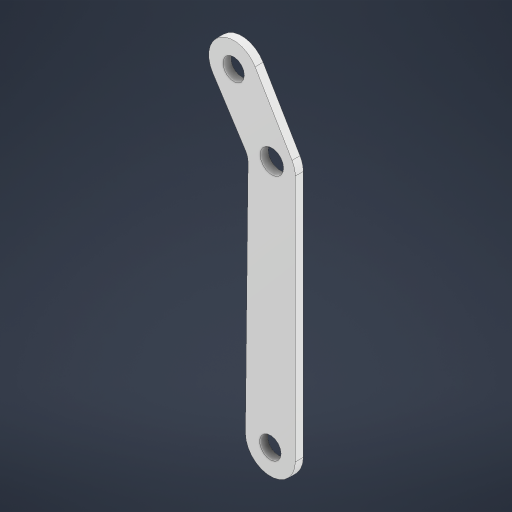
# Autodesk Inventor part: pneumaticwingplexi
Saved by Autodesk Inventor 2023 (Build 270158000, 158)
## iProperties
Created: 2023-08-07
Part Number: pneumaticwingplexi
Material: Generic
Document SubType Name: Modeling
Designer: srbel
Density: 1 g/cm^3
Appearance: Smooth - White
Mass: 1.20002 g
Surface Area: 18.206 cm^2
Volume: 1.20002 cm^3
Author: srbel
Autodesk Inventor part; units mm, degrees
ref_plane "YZ Plane" through (0, 0, 0) normal (1, 0, 0) x (0, 1, 0)
ref_plane "XZ Plane" through (0, 0, 0) normal (0, 1, 0) x (-1, 0, 0)
ref_plane "XY Plane" through (0, 0, 0) normal (0, 0, 1) x (1, 0, 0)
sketch "Sketch2" plane through (0, 0, 0) normal (0, 0, 1) x (1, 0, 0)
  circle A0 centre (-4.7681, 50.6628) radius 2.39
  circle A1 centre (-4.7681, 50.6628) radius 2.39
  circle A2 centre (-5.08, 0) radius 2.1844
  circle A3 centre (-12.5662, 63.0568) radius 2.1844
  arc A4 (-10.1597, 0.0569) -> (0, 0) centre (-5.08, 0) ccw
  arc A5 (-8.1919, 65.6399) -> (-16.8387, 60.3087) centre (-12.5662, 63.0568) ccw
  line L0 (-16.8387, 60.3087) -> (-10.1261, 49.8724)
  line L1 (-0.6665, 52.8961) -> (-8.1919, 65.6399)
  line L2 (0, 0) -> (0, 50.4566)
  arc A6 (0, 50.4566) -> (-0.6665, 52.8961) centre (-4.7976, 50.4566) ccw
  line L3 (-9.6216, 48.1193) -> (-10.1597, 0.0569)
  arc A7 (-9.6216, 48.1193) -> (-10.1261, 49.8724) centre (-12.7964, 48.1549) ccw
  circle A8 centre (-12.5662, 63.0568) radius 2.1844
  circle A9 centre (-5.08, 0) radius 2.1844
  arc A10 (-10.1597, 0.0569) -> (0, 0) centre (-5.08, 0) ccw
  line L4 (-10.1597, 0.0569) -> (-9.6216, 48.1193)
  line L5 (-10.1261, 49.8724) -> (-16.8387, 60.3087)
  arc A11 (-9.6216, 48.1193) -> (-10.1261, 49.8724) centre (-12.7964, 48.1549) ccw
  arc A12 (-8.1919, 65.6399) -> (-16.8387, 60.3087) centre (-12.5662, 63.0568) ccw
  line L6 (-8.1919, 65.6399) -> (-0.6665, 52.8961)
  constraints: 14 end point, 14 point on circle, 13 centre point, 6 concentric, 5 coincident, 3 collinear, 3 tangent
extrude "Extrusion4" add sketch "Sketch2" along normal blind 1.62
body "Solid4"
